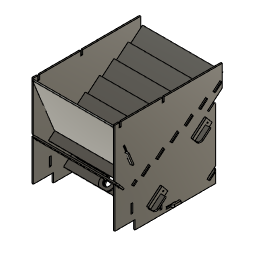
Lego Feeder (Autodesk Fusion 360 design; units mm, degrees)
Autodesk Fusion 360 part; units mm, degrees
sketch "Sketch2" plane through (0, 0, 0) normal (0, 0, 1) x (1, 0, 0) in component "SidePanel"
  line L0 (-258.4316, 256.8054) -> (-243.1107, 269.6612)
  line L1 (-243.1107, 269.6612) -> (-245.0391, 271.9593)
  line L2 (-260.36, 259.1035) -> (-245.0391, 271.9593)
  line L3 (-258.4316, 256.8054) -> (-260.36, 259.1035)
  line L4 (-228.4061, 275.4727) -> (-213.0852, 288.3285)
  line L5 (-226.4778, 273.1746) -> (-228.4061, 275.4727)
  line L6 (-211.1569, 286.0304) -> (-213.0852, 288.3285)
  line L7 (-226.4778, 273.1746) -> (-211.1569, 286.0304)
  line L8 (-164.4984, 308.2112) -> (-149.1775, 321.0669)
  line L9 (-162.5701, 305.913) -> (-164.4984, 308.2112)
  line L10 (-162.5701, 305.913) -> (-147.2492, 318.7688)
  line L11 (-147.2492, 318.7688) -> (-149.1775, 321.0669)
  line L12 (-196.4523, 291.842) -> (-181.1314, 304.6977)
  line L13 (-194.5239, 289.5438) -> (-196.4523, 291.842)
  line L14 (-179.203, 302.3996) -> (-181.1314, 304.6977)
  line L15 (-194.5239, 289.5438) -> (-179.203, 302.3996)
  line L16 (-132.5446, 324.5804) -> (-117.2237, 337.4361)
  line L17 (-130.6162, 322.2822) -> (-132.5446, 324.5804)
  line L18 (-115.2953, 335.138) -> (-117.2237, 337.4361)
  line L19 (-130.6162, 322.2822) -> (-115.2953, 335.138)
  line L20 (-100.5907, 340.9496) -> (-85.2698, 353.8053)
  line L21 (-98.6623, 338.6515) -> (-100.5907, 340.9496)
  line L22 (-83.3414, 351.5072) -> (-85.2698, 353.8053)
  line L23 (-98.6623, 338.6515) -> (-83.3414, 351.5072)
  line L24 (-320, 385) -> (-310, 385)
  line L25 (-310, 385) -> (-310, 375)
  line L26 (-310, 375) -> (-306, 375)
  line L27 (-306, 375) -> (-306, 385)
  line L28 (-214, 385) -> (-214, 375)
  line L29 (-214, 375) -> (-210, 375)
  line L30 (-210, 375) -> (-210, 385)
  line L31 (-306, 385) -> (-214, 385)
  line L32 (-210, 385) -> (-80, 385)
  line L33 (-270, 160) -> (-95, 160)
  line L34 (-270, 160) -> (-275, 160)
  line L35 (-275, 160) -> (-275, 180)
  line L36 (-320, 180) -> (-275, 180)
  line L37 (-110.3209, 306.5578) -> (-112.892, 309.6219)
  line L38 (-112.892, 309.6219) -> (-80, 337.2216)
  line L39 (-320, 270) -> (-310.3582, 258.5093)
  line L40 (-310.3582, 258.5093) -> (-307.294, 261.0805)
  line L41 (-307.294, 261.0805) -> (-320, 276.2229)
  line L42 (-110.3209, 306.5578) -> (-98.8302, 316.1996)
  arc A0 (-95, 314.5191) -> (-98.8302, 316.1996) centre (-97.3306, 314.4124) ccw
  line L43 (-245.0047, 186.3535) -> (-242.4335, 183.2893)
  line L44 (-245.0047, 186.3535) -> (-222.0233, 205.6371)
  line L45 (-242.4335, 183.2893) -> (-219.4522, 202.5729)
  line L46 (-219.4522, 202.5729) -> (-222.0233, 205.6371)
  line L47 (-122.4376, 289.1995) -> (-119.8664, 286.1353)
  line L48 (-122.4376, 289.1995) -> (-145.4189, 269.9158)
  line L49 (-119.8664, 286.1353) -> (-142.8477, 266.8517)
  line L50 (-142.8477, 266.8517) -> (-145.4189, 269.9158)
  line L51 (-80, 337.2216) -> (-80, 385)
  line L52 (-95, 160) -> (-95, 189)
  line L53 (-95, 194.2216) -> (-95, 314.5191)
  line L54 (-95, 189) -> (-106.4907, 179.3582)
  line L55 (-106.4907, 179.3582) -> (-109.0618, 182.4224)
  line L56 (-109.0618, 182.4224) -> (-95, 194.2216)
  line L57 (-272.7665, 255.2203) -> (-274.6948, 257.5184)
  line L58 (-272.7665, 255.2203) -> (-280.4269, 248.7924)
  line L59 (-274.6948, 257.5184) -> (-282.3553, 251.0906)
  line L60 (-280.4269, 248.7924) -> (-282.3553, 251.0906)
  line L61 (-320, 180) -> (-320, 270)
  line L62 (-320, 276.2229) -> (-320, 385)
  line L63 (-280, 195) -> (-284, 195)
  line L64 (-284, 195) -> (-284, 215)
  line L65 (-284, 215) -> (-280, 215)
  line L66 (-280, 215) -> (-280, 195)
  line L67 (-287.3826, 307.9489) -> (-298.1337, 335.9564)
  line L68 (-287.3826, 307.9489) -> (-290.1834, 306.8738)
  line L69 (-290.1834, 306.8738) -> (-300.9344, 334.8813)
  line L70 (-300.9344, 334.8813) -> (-298.1337, 335.9564)
  line L71 (-219, 170) -> (-219, 190)
  line L72 (-219, 190) -> (-215, 190)
  line L73 (-215, 190) -> (-215, 170)
  line L74 (-215, 170) -> (-219, 170)
  line L75 (-185, 165) -> (-205, 165)
  line L76 (-205, 165) -> (-205, 170)
  line L77 (-205, 170) -> (-185, 170)
  line L78 (-185, 170) -> (-185, 165)
  dimension "d102_1" = 20
  dimension "d107_1" = 20
  dimension "d109_1" = 20
  dimension "d111_1" = 20
  dimension "d113_1" = 20
  dimension "d115_1" = 20
  dimension "d2" = 4
  dimension "d3" = 15
  dimension "d4" = 15
  dimension "d104" = 4
  dimension "d110" = 4
  dimension "d112" = 30
  dimension "d118" = 15
  dimension "d119" = 4
  dimension "d134" = 10
  dimension "d163" = 3
  dimension "d164" = 30
  dimension "d165" = 20
  dimension "d166" = 5
  constraint perpendicular L0 L1
  constraint perpendicular L2 L3
  constraint perpendicular L6 L7
  constraint perpendicular L4 L5
  constraint perpendicular L14 L15
  constraint perpendicular L12 L13
  constraint perpendicular L10 L11
  constraint perpendicular L8 L9
  constraint perpendicular L18 L19
  constraint perpendicular L16 L17
  constraint perpendicular L22 L23
  constraint perpendicular L20 L21
  constraint perpendicular L24 L25
  constraint perpendicular L25 L26
  constraint perpendicular L27 L29
  constraint perpendicular L28 L31
  constraint perpendicular L37 L38
  constraint perpendicular L39 L40
  constraint perpendicular L40 L41
  constraint perpendicular L37 L42
  constraint tangent L42 A0
  constraint perpendicular L43 L44
  constraint perpendicular L43 L45
  constraint perpendicular L47 L48
  constraint perpendicular L47 L49
  constraint perpendicular L33 L52
  constraint perpendicular L54 L55
  constraint perpendicular L55 L56
  constraint perpendicular L57 L58
  constraint perpendicular L57 L59
  constraint perpendicular L59 L60
  constraint perpendicular L24 L62
  constraint horizontal L63
  constraint vertical L64
  constraint horizontal L65
  constraint vertical L66
  constraint perpendicular L67 L68
  constraint perpendicular L68 L69
  constraint horizontal L74
  constraint vertical L71
  constraint horizontal L72
  constraint vertical L73
  constraint horizontal L75
  constraint vertical L76
  constraint horizontal L77
  constraint vertical L78
  measures "d102_1" distance of L0.start L0.end
  measures "d107_1" distance of L6.start L5.start
  measures "d109_1" distance of L13.start L14.start
  measures "d111_1" distance of L9.start L10.end
  measures "d113_1" distance of L18.start L17.start
  measures "d115_1" distance of L21.start L22.start
  measures "d2" distance of L37.start L37.end
  measures "d3" distance of L39.start L39.end
  measures "d4" distance of L37.start L42.end
  measures "d104" distance of L43.start L43.end
  measures "d110" distance of L47.start L47.end
  measures "d112" distance of L47.end L49.end
  measures "d118" distance of L52.end L54.end
  measures "d119" distance of L54.end L55.end
  measures "d134" distance of L57.end L59.end
  measures "d163" distance of L67.start L68.end
  measures "d164" distance of L68.end L69.end
  measures "d165" distance of L75.start L75.end
  measures "d166" distance of L75.start L77.end
sketch "Sketch1" plane through (0, 0, 0) normal (0, 0, 1) x (1, 0, 0) in component "BackWall"
  line L0 (-315, 105) -> (-318, 105)
  line L1 (-315, 105) -> (-315, 55)
  line L2 (-315, 55) -> (-136, 55)
  line L3 (-136, 55) -> (-136, 105)
  line L4 (-318, 105) -> (-318, 90)
  line L5 (-315, 120) -> (-315, 185)
  line L6 (-315, 185) -> (-136, 185)
  line L7 (-136, 185) -> (-136, 120)
  line L8 (-133, 90) -> (-133, 105)
  line L9 (-133, 105) -> (-136, 105)
  line L10 (-318, 90) -> (-324, 90)
  line L11 (-324, 90) -> (-324, 120)
  line L12 (-324, 120) -> (-315, 120)
  line L13 (-133, 90) -> (-127, 90)
  line L14 (-127, 90) -> (-127, 120)
  line L15 (-127, 120) -> (-136, 120)
  dimension "d143" = 50
  dimension "d144" = 179
  dimension "d145" = 15
  dimension "d148" = 65
  constraint perpendicular L0 L1
  constraint perpendicular L2 L3
  constraint perpendicular L0 L4
  constraint perpendicular L5 L6
  constraint perpendicular L6 L7
  constraint perpendicular L4 L10
  constraint perpendicular L10 L11
  constraint perpendicular L5 L12
  constraint perpendicular L7 L15
  measures "d143" distance of L0.start L1.end
  measures "d144" distance of L1.end L2.end
  measures "d145" distance of L0.end L4.end
  measures "d148" distance of L5.start L5.end
extrude "Extrude1" add sketch "Sketch2" along normal blind 3 makes body 1 in component "SidePanel"
sketch "Sketch1 (2)" plane through (0, 0, 0) normal (0, 0, 1) x (1, 0, 0) in component "Step"
  line L0 (25, 360) -> (204, 360)
  line L1 (204, 403) -> (25, 403)
  line L2 (25, 403) -> (25, 393)
  line L3 (25, 373) -> (25, 360)
  line L4 (204, 403) -> (204, 393)
  line L5 (204, 373) -> (204, 360)
  line L6 (25, 373) -> (19, 373)
  line L7 (19, 373) -> (19, 393)
  line L8 (19, 393) -> (25, 393)
  line L9 (204, 373) -> (210, 373)
  line L10 (210, 373) -> (210, 393)
  line L11 (210, 393) -> (204, 393)
  dimension "d5" = 179
  dimension "d6" = 43
  dimension "d7" = 10
  dimension "d10" = 10
  dimension "d204" = 6
  dimension "d205" = 20
  constraint horizontal L0
  constraint horizontal L1
  constraint perpendicular L1 L2
  constraint perpendicular L1 L4
  constraint perpendicular L0 L5
  constraint perpendicular L3 L6
  constraint perpendicular L6 L7
  constraint perpendicular L9 L10
  measures "d5" distance of L0.start L0.end
  measures "d6" distance of L0.start L1.end
  measures "d7" distance of L1.end L2.end
  measures "d10" distance of L1.start L4.end
  measures "d204" distance of L3.start L6.end
  measures "d205" distance of L6.end L7.end
sketch "Sketch1 (3)" plane through (0, 0, 0) normal (0, 0, 1) x (1, 0, 0) in component "LastStep"
  line L0 (25, 423) -> (25, 410)
  line L1 (25, 410) -> (204, 410)
  line L2 (204, 423) -> (204, 410)
  line L3 (25, 443) -> (25, 448)
  line L4 (25, 448) -> (204, 448)
  line L5 (204, 448) -> (204, 443)
  line L6 (204, 423) -> (210, 423)
  line L7 (210, 423) -> (210, 443)
  line L8 (210, 443) -> (204, 443)
  line L9 (25, 423) -> (19, 423)
  line L10 (19, 423) -> (19, 443)
  line L11 (19, 443) -> (25, 443)
  dimension "d11" = 179
  dimension "d206" = 6
  constraint horizontal L1
  constraint perpendicular L1 L2
  constraint perpendicular L6 L7
  constraint perpendicular L0 L9
  measures "d11" distance of L1.end L0.end
  measures "d206" distance of L0.start L9.end
sketch "Sketch1 (4)" plane through (0, 0, 0) normal (0, 0, 1) x (1, 0, 0) in component "MovingStep"
  line L0 (26, 355) -> (203, 355)
  circle A0 centre (90, 265) radius 1.5
  circle A1 centre (139, 265) radius 1.5
  circle A2 centre (114.5, 265) radius 4
  arc A3 (146, 258) -> (153, 265) centre (146, 265) ccw
  line L1 (146, 258) -> (83, 258)
  arc A4 (76, 265) -> (83, 258) centre (83, 265) ccw
  line L2 (153, 265) -> (153, 300)
  arc A5 (160, 307) -> (153, 300) centre (160, 300) ccw
  line L3 (76, 265) -> (76, 300)
  arc A6 (76, 300) -> (69, 307) centre (69, 300) ccw
  line L4 (160, 307) -> (196, 307)
  line L5 (203, 355) -> (203, 314)
  arc A7 (196, 307) -> (203, 314) centre (196, 314) ccw
  line L6 (69, 307) -> (33, 307)
  line L7 (26, 355) -> (26, 314)
  arc A8 (26, 314) -> (33, 307) centre (33, 314) ccw
  circle A9 centre (139, 300) radius 2.6
  circle A10 centre (90, 300) radius 2.6
  circle A11 centre (114.5, 300) radius 6
  dimension "d26" = 3
  dimension "d27" = 8
  dimension "d32" = 63
  dimension "d33" = 35
  dimension "d36" = 35
  dimension "d37" = 36
  dimension "d38" = 41
  dimension "d39" = 36
  dimension "d40" = 41
  dimension "d181" = 5.2
  dimension "d182" = 5.2
  dimension "d203" = 12
  constraint horizontal L0
  constraint tangent L2 A5
  constraint vertical L3
  constraint tangent L3 A6
  constraint perpendicular L0 L5
  constraint tangent L5 A7
  constraint tangent L4 A7
  constraint perpendicular L0 L7
  constraint tangent L7 A8
  measures "d26" diameter of A1
  measures "d27" diameter of A2
  measures "d32" distance of A3.start L1.end
  measures "d33" distance of A3.end L2.end
  measures "d36" distance of A4.start L3.end
  measures "d37" distance of A5.start L4.end
  measures "d38" distance of L0.end L5.end
  measures "d39" distance of A6.end L6.end
  measures "d40" distance of L0.start L7.end
  measures "d181" diameter of A9
  measures "d182" diameter of A10
  measures "d203" diameter of A11
sketch "Sketch1 (5)" plane through (0, 0, 0) normal (0, 0, 1) x (1, 0, 0) in component "StepSpacer"
  circle A0 centre (139, 249) radius 1.5
  circle A1 centre (90, 249) radius 1.5
  circle A2 centre (114.5, 249) radius 4
  arc A3 (83, 256) -> (83, 242) centre (83, 249) ccw
  arc A4 (146, 242) -> (146, 256) centre (146, 249) ccw
  line L0 (83, 256) -> (146, 256)
  line L1 (146, 242) -> (83, 242)
  dimension "d41" = 3
  dimension "d42" = 8
  constraint tangent A4 L0
  constraint tangent A3 L1
  measures "d41" diameter of A0
  measures "d42" diameter of A2
sketch "Sketch2 (2)" plane through (0, 0, 0) normal (0, 0, 1) x (1, 0, 0) in component "MovingStepFirst"
  arc A0 (340, 307) -> (333, 300) centre (340, 300) ccw
  line L0 (383, 355) -> (383, 314)
  line L1 (249, 307) -> (213, 307)
  line L2 (340, 307) -> (376, 307)
  arc A1 (206, 314) -> (213, 307) centre (213, 314) ccw
  line L3 (206, 355) -> (206, 314)
  line L4 (206, 355) -> (383, 355)
  arc A2 (256, 300) -> (249, 307) centre (249, 300) ccw
  arc A3 (376, 307) -> (383, 314) centre (376, 314) ccw
  arc A4 (326, 293) -> (333, 300) centre (326, 300) ccw
  arc A5 (256, 300) -> (263, 293) centre (263, 300) ccw
  line L5 (263, 293) -> (326, 293)
  circle A6 centre (319, 300) radius 2.6
  circle A7 centre (270, 300) radius 2.6
  dimension "d61" = 36
  dimension "d62" = 41
  dimension "d63" = 36
  dimension "d64" = 41
  dimension "d183" = 5.2
  dimension "d184" = 5.2
  constraint horizontal L4
  constraint perpendicular L0 L4
  constraint tangent L0 A3
  constraint tangent L2 A3
  constraint perpendicular L3 L4
  constraint tangent A1 L3
  constraint tangent A4 L5
  measures "d61" distance of A0.start L2.end
  measures "d62" distance of L0.start L0.end
  measures "d63" distance of L1.start L1.end
  measures "d64" distance of A1.start L3.start
  measures "d183" diameter of A6
  measures "d184" diameter of A7
sketch "Sketch1 (6)" plane through (0, 0, 0) normal (0, 0, 1) x (1, 0, 0) in component "Brace"
  line L0 (25, 215) -> (204, 215)
  line L1 (204, 215) -> (204, 225)
  line L2 (204, 225) -> (207, 225)
  line L3 (207, 225) -> (207, 215)
  line L4 (207, 215) -> (211, 215)
  line L5 (25, 215) -> (25, 225)
  line L6 (25, 225) -> (22, 225)
  line L7 (22, 225) -> (22, 215)
  line L8 (22, 215) -> (18, 215)
  line L9 (211, 215) -> (211, 231)
  arc A0 (211, 231) -> (207, 235) centre (207, 231) ccw
  line L10 (18, 215) -> (18, 231)
  line L11 (207, 235) -> (22, 235)
  arc A1 (22, 235) -> (18, 231) centre (22, 231) ccw
  dimension "d65" = 179
  constraint horizontal L0
  constraint perpendicular L0 L1
  constraint perpendicular L1 L2
  constraint perpendicular L2 L3
  constraint perpendicular L3 L4
  constraint perpendicular L0 L5
  constraint perpendicular L5 L6
  constraint perpendicular L0 L7
  constraint perpendicular L7 L8
  constraint perpendicular L4 L9
  constraint tangent L9 A0
  constraint perpendicular L8 L10
  constraint horizontal L11
  constraint tangent L10 A1
  measures "d65" distance of L0.start L0.end
extrude "Extrude1'" add sketch "Sketch1 (4)" along normal blind 4 separate body contours L0 A3 L1 A4 L2 A5 L3 A6 L4 L5 A7 L6 L7 A8 | A11 makes body 2 in component "MovingStep"
extrude "Extrude1''" add sketch "Sketch1 (5)" along normal blind 4 separate body makes body 3 in component "StepSpacer"
extrude "Extrude1'''" add sketch "Sketch2 (2)" along normal blind 4 separate body makes body 4 in component "MovingStepFirst"
extrude "Extrude1''''" add sketch "Sketch1 (2)" along normal blind 3 separate body makes body 5 in component "Step"
extrude "Extrude1'''''" add sketch "Sketch1 (3)" along normal blind 3 separate body makes body 6 in component "LastStep"
sketch "Sketch1 (7)" plane through (0, 0, 0) normal (0, 0, 1) x (1, 0, 0) in component "Mount"
  line L0 (25, 205) -> (204, 205)
  line L1 (204, 25) -> (25, 25)
  circle A0 centre (129.5, 100) radius 1.5
  circle A1 centre (99.5, 100) radius 1.5
  circle A2 centre (99.5, 130) radius 1.5
  circle A3 centre (129.5, 130) radius 1.5
  circle A4 centre (114.5, 122) radius 6.5
  line L2 (25, 25) -> (25, 35)
  line L3 (204, 195) -> (204, 205)
  line L4 (204, 25) -> (204, 35)
  arc A5 (204, 155) -> (204, 75) centre (204, 115) ccw
  line L5 (204, 65) -> (204, 75)
  line L6 (204, 155) -> (204, 165)
  line L7 (25, 195) -> (25, 205)
  line L8 (25, 165) -> (25, 155)
  line L9 (25, 65) -> (25, 75)
  arc A6 (25, 75) -> (25, 155) centre (25, 115) ccw
  arc A7 (108, 143) -> (121, 143) centre (114.5, 143) ccw
  arc A8 (121, 192) -> (108, 192) centre (114.5, 192) ccw
  arc A9 (121, 87) -> (108, 87) centre (114.5, 87) ccw
  arc A10 (108, 38) -> (121, 38) centre (114.5, 38) ccw
  line L10 (108, 38) -> (108, 87)
  line L11 (121, 38) -> (121, 87)
  line L12 (108, 143) -> (108, 192)
  line L13 (121, 143) -> (121, 192)
  circle A11 centre (127, 84) radius 1.5
  circle A12 centre (102, 84) radius 1.5
  circle A13 centre (102, 41) radius 1.5
  circle A14 centre (127, 41) radius 1.5
  circle A15 centre (127, 146) radius 1.5
  circle A16 centre (102, 146) radius 1.5
  circle A17 centre (102, 189) radius 1.5
  circle A18 centre (127, 189) radius 1.5
  line L14 (204, 65) -> (206.8, 65)
  line L15 (206.8, 35) -> (204, 35)
  line L16 (211.2, 65) -> (211.2, 55)
  line L17 (211.2, 55) -> (206.8, 55)
  line L18 (211.2, 65) -> (221.2, 65)
  arc A19 (214.2, 35) -> (221.2, 42) centre (214.2, 42) ccw
  line L19 (206.8, 35) -> (214.2, 35)
  line L20 (221.2, 42) -> (221.2, 65)
  line L21 (206.8, 55) -> (206.8, 65)
  line L22 (221.2, 172) -> (221.2, 195)
  line L23 (211.2, 195) -> (211.2, 185)
  arc A20 (214.2, 165) -> (221.2, 172) centre (214.2, 172) ccw
  line L24 (206.8, 165) -> (214.2, 165)
  line L25 (206.8, 185) -> (206.8, 195)
  line L26 (211.2, 185) -> (206.8, 185)
  line L27 (211.2, 195) -> (221.2, 195)
  line L28 (206.8, 195) -> (204, 195)
  line L29 (206.8, 165) -> (204, 165)
  line L30 (7.8, 42) -> (7.8, 65)
  line L31 (17.8, 65) -> (17.8, 55)
  arc A21 (14.8, 35) -> (7.8, 42) centre (14.8, 42) cw
  line L32 (22.2, 35) -> (14.8, 35)
  line L33 (22.2, 55) -> (22.2, 65)
  line L34 (17.8, 55) -> (22.2, 55)
  line L35 (17.8, 65) -> (7.8, 65)
  line L36 (22.2, 65) -> (25, 65)
  line L37 (22.2, 35) -> (25, 35)
  line L38 (17.8, 65) -> (17.8, 55)
  line L39 (22.2, 55) -> (22.2, 65)
  line L40 (17.8, 55) -> (22.2, 55)
  line L41 (22.2, 35) -> (14.8, 35)
  line L42 (17.8, 65) -> (7.8, 65)
  arc A22 (14.8, 35) -> (7.8, 42) centre (14.8, 42) cw
  line L43 (7.8, 42) -> (7.8, 65)
  line L44 (17.8, 195) -> (17.8, 185)
  line L45 (22.2, 185) -> (22.2, 195)
  line L46 (17.8, 185) -> (22.2, 185)
  line L47 (22.2, 165) -> (14.8, 165)
  line L48 (17.8, 195) -> (7.8, 195)
  arc A23 (14.8, 165) -> (7.8, 172) centre (14.8, 172) cw
  line L49 (7.8, 172) -> (7.8, 195)
  line L50 (22.2, 195) -> (25, 195)
  line L51 (22.2, 165) -> (25, 165)
  dimension "d85" = 179
  dimension "d86" = 180
  dimension "d185" = 2.8
  dimension "d187" = 10
  dimension "d190" = 10
  dimension "d191" = 10
  dimension "d192" = 10
  dimension "d193" = 10
  constraint horizontal L0
  constraint horizontal L1
  constraint perpendicular L0 L3
  constraint perpendicular L0 L7
  constraint tangent A9 L10
  constraint tangent A9 L11
  constraint tangent A8 L12
  constraint perpendicular L5 L14
  constraint perpendicular L16 L18
  constraint tangent A19 L19
  constraint tangent A19 L20
  constraint perpendicular L14 L21
  constraint perpendicular L23 L27
  constraint tangent A20 L24
  constraint tangent L22 A20
  constraint perpendicular L31 L35
  constraint tangent A21 L32
  constraint tangent L30 A21
  constraint perpendicular L9 L36
  constraint perpendicular L38 L42
  constraint tangent L41 A22
  constraint tangent A22 L43
  constraint perpendicular L44 L48
  constraint tangent L47 A23
  constraint tangent A23 L49
  measures "d85" distance of L0.start L0.end
  measures "d86" distance of L0.start L1.end
  measures "d185" distance of L5.start L14.end
  measures "d187" distance of L16.start L18.end
  measures "d190" distance of L23.start L22.end
  measures "d191" distance of L31.start L30.end
  measures "d192" distance of L31.start L30.end
  measures "d193" distance of L44.start L48.end
extrude "Extrude2" add sketch "Sketch1 (7)" along normal blind 4 separate body makes body 7 in component "Mount"
sketch "Sketch1 (8)" plane through (0, 0, 0) normal (0, 0, 1) x (1, 0, 0) in component "BearingGuide"
  line L0 (242.941, 100) -> (226.059, 100)
  arc A0 (226.059, 100) -> (219, 87) centre (234.5, 87) ccw
  line L1 (219, 38) -> (219, 87)
  arc A1 (219, 38) -> (226.059, 25) centre (234.5, 38) ccw
  line L2 (226.059, 25) -> (242.941, 25)
  arc A2 (242.941, 25) -> (250, 38) centre (234.5, 38) ccw
  line L3 (250, 38) -> (250, 87)
  arc A3 (250, 87) -> (242.941, 100) centre (234.5, 87) ccw
  circle A4 centre (247, 41) radius 1.5
  circle A5 centre (222, 41) radius 1.5
  circle A6 centre (222, 84) radius 1.5
  circle A7 centre (247, 84) radius 1.5
  arc A8 (226.25, 38) -> (242.75, 38) centre (234.5, 38) ccw
  arc A9 (242.75, 87) -> (226.25, 87) centre (234.5, 87) ccw
  line L4 (226.25, 38) -> (226.25, 87)
  line L5 (242.75, 38) -> (242.75, 87)
  dimension "d196" = 8.25
  dimension "d197" = 8.25
  constraint tangent L3 A3
  constraint tangent A0 L1
  constraint coincident A0.centre A3.centre
  constraint tangent A9 L4
  constraint tangent A9 L5
  measures "d196" radius of A8
  measures "d197" radius of A9
extrude "Extrude1''''''" add sketch "Sketch1 (8)" along normal blind 3 separate body makes body 8 in component "BearingGuide"
extrude "Extrude1'''''''" add sketch "Sketch1 (6)" along normal blind 3 separate body makes body 9 in component "Brace"
sketch "Sketch2 (3)" plane through (0, 0, 0) normal (0, 0, 1) x (1, 0, 0) in component "FirstStep"
  line L0 (25, 453) -> (204, 453)
  line L1 (25, 473) -> (204, 473)
  line L2 (204, 473) -> (204, 468)
  line L3 (25, 453) -> (25, 458)
  line L4 (204, 453) -> (204, 458)
  line L5 (25, 473) -> (25, 468)
  line L6 (25, 458) -> (19, 458)
  line L7 (19, 458) -> (19, 468)
  line L8 (19, 468) -> (25, 468)
  line L9 (204, 458) -> (210, 458)
  line L10 (210, 458) -> (210, 468)
  line L11 (210, 468) -> (204, 468)
  dimension "d126" = 179
  dimension "d129" = 5
  dimension "d207" = 6
  dimension "d208" = 10
  constraint horizontal L0
  constraint perpendicular L1 L5
  constraint perpendicular L3 L6
  constraint perpendicular L6 L7
  constraint perpendicular L4 L9
  constraint perpendicular L9 L10
  measures "d126" distance of L0.end L0.start
  measures "d129" distance of L1.start L5.end
  measures "d207" distance of L3.end L6.end
  measures "d208" distance of L6.end L7.end
extrude "Extrude1''''''''" add sketch "Sketch2 (3)" along normal blind 3 separate body makes body 10 in component "FirstStep"
extrude "Extrude1'''''''''" add sketch "Sketch1" along normal blind 3 separate body makes body 11 in component "BackWall"
sketch "Sketch1 (9)" plane through (0, 0, 0) normal (0, 0, 1) x (1, 0, 0) in component "MotorArm"
  arc A0 (261.2507, 33.25) -> (264.7493, 33.25) centre (263, 31) ccw
  circle A1 centre (285.5, 31) radius 2
  arc A2 (263, 38) -> (263, 24) centre (263, 31) ccw
  arc A3 (285.5, 24) -> (285.5, 38) centre (285.5, 31) ccw
  line L0 (263, 33.25) -> (264.7493, 33.25)
  line L1 (263, 33.25) -> (261.2507, 33.25)
  line L2 (263, 38) -> (285.5, 38)
  line L3 (285.5, 24) -> (263, 24)
  constraint coincident A1.centre A3.centre
  constraint coincident A0.centre A2.centre
  constraint tangent A2 L3
sketch "Sketch1 (10)" plane through (0, 0, 0) normal (0, 0, 1) x (1, 0, 0) in component "LinkArm"
  circle A0 centre (260, 10) radius 2.25
  circle A1 centre (319.5, 10) radius 4.25
  arc A2 (260, 17) -> (260, 3) centre (260, 10) ccw
  arc A3 (319.5, 0) -> (319.5, 20) centre (319.5, 10) ccw
  line L0 (319.5, 0) -> (260, 3)
  line L1 (260, 17) -> (319.5, 20)
  dimension "d171" = 4.5
  dimension "d172" = 59.5
  dimension "d173" = 8.5
  dimension "d175" = 7
  dimension "d176" = 10
  constraint coincident A0.centre A2.centre
  constraint coincident A1.centre A3.centre
  measures "d171" diameter of A0
  measures "d172" distance of A0.centre A1.centre
  measures "d173" diameter of A1
  measures "d175" radius of A2
  measures "d176" radius of A3
extrude "Extrude1''''''''''" add sketch "Sketch1 (10)" along normal blind 4 separate body makes body 12 in component "LinkArm"
extrude "Extrude1'''''''''''" add sketch "Sketch1 (9)" along normal blind 4 separate body makes body 13 in component "MotorArm"
sketch "Sketch1 (11)" plane through (0, 0, 0) normal (0, 0, 1) x (1, 0, 0) in component "LockingPiece"
  line L0 (273, 75) -> (273, 55)
  line L1 (273, 55) -> (265, 55)
  line L2 (285, 55) -> (277, 55)
  line L3 (277, 55) -> (277, 75)
  line L4 (285, 95) -> (265, 95)
  line L5 (273, 75) -> (277, 75)
  line L6 (265, 55) -> (265, 95)
  line L7 (285, 55) -> (285, 95)
  circle A0 centre (275, 90) radius 1.5
  dimension "d200" = 3
  constraint vertical L0
  constraint horizontal L1
  constraint horizontal L2
  constraint vertical L3
  constraint horizontal L4
  constraint perpendicular L0 L5
  constraint perpendicular L4 L6
  measures "d200" diameter of A0
extrude "Extrude1''''''''''''" add sketch "Sketch1 (11)" along normal blind 4 separate body makes body 14 in component "LockingPiece"
sketch "Sketch 1" plane through (0, 0, 0) normal (0, 0, 1) x (1, 0, 0) in component "Power supply holder"
  line L0 (-71, 19) -> (-68, 19)
  line L1 (-42, -13) -> (-64, -13)
  arc A0 (-38, -9) -> (-42, -13) centre (-42, -9) cw
  arc A1 (-64, -13) -> (-68, -9) centre (-64, -9) cw
  line L2 (-68, -9) -> (-68, 10)
  circle A2 centre (-64, 38) radius 1.25
  arc A3 (-42, 42) -> (-38, 38) centre (-42, 38) cw
  arc A4 (-75, 15) -> (-71, 19) centre (-71, 15) cw
  line L3 (-68, 19) -> (-68, 38)
  line L4 (-71, 10) -> (-71, 0)
  circle A5 centre (-42, 38) radius 1.25
  line L5 (-38, 38) -> (-38, -9)
  line L6 (-64, 42) -> (-42, 42)
  arc A6 (-68, 38) -> (-64, 42) centre (-64, 38) cw
  line L7 (-68, 10) -> (-71, 10)
  line L8 (-71, 0) -> (-75, 0)
  line L9 (-75, 0) -> (-75, 15)
  circle A7 centre (-64, -9) radius 1.25
  circle A8 centre (-42, -9) radius 1.25
extrude "Extrude1'''''''''''''" add sketch "Sketch 1" along normal blind 5 separate body makes body 15 in component "Power supply holder"
component "Templates" placed x (1, 0, 0) y (0, 1, 0) z (0, 0, 1) at (0, 0, 0)
component "LegoFeeder" placed x (1, 0, 0) y (0, 1, 0) z (0, 0, 1) at (0, 0, 0)
component "SidePanel" placed x (1, 0, 0) y (0, 1, 0) z (0, 0, 1) at (0, 0, 0) in component "Templates"
component "BackWall" placed x (1, 0, 0) y (0, 1, 0) z (0, 0, 1) at (0, -50, 0) in component "Templates"
component "Step" placed x (1, 0, 0) y (0, 1, 0) z (0, 0, 1) at (0, 0, 0) in component "Templates"
component "LastStep" placed x (1, 0, 0) y (0, 1, 0) z (0, 0, 1) at (0, 0, 0) in component "Templates"
component "MovingStep" placed x (1, 0, 0) y (0, 1, 0) z (0, 0, 1) at (0, 0, 0) in component "Templates"
component "StepSpacer" placed x (1, 0, 0) y (0, 1, 0) z (0, 0, 1) at (0, 0, 0) in component "Templates"
component "MovingStepFirst" placed x (1, 0, 0) y (0, 1, 0) z (0, 0, 1) at (0, 0, 0) in component "Templates"
component "Brace" placed x (1, 0, 0) y (0, 1, 0) z (0, 0, 1) at (0, 0, 0) in component "Templates"
component "Mount" placed x (1, 0, 0) y (0, 1, 0) z (0, 0, 1) at (0, 0, 0) in component "Templates"
component "BearingGuide" placed x (1, 0, 0) y (0, 1, 0) z (0, 0, 1) at (0, 0, 0) in component "Templates"
component "FirstStep" placed x (1, 0, 0) y (0, 1, 0) z (0, 0, 1) at (0, 0, 0) in component "Templates"
component "MotorArm" placed x (1, 0, 0) y (0, 1, 0) z (0, 0, 1) at (0, 0, 0) in component "Templates"
component "LinkArm" placed x (1, 0, 0) y (0, 1, 0) z (0, 0, 1) at (0, 0, 0) in component "Templates"
component "LockingPiece" placed x (1, 0, 0) y (0, 1, 0) z (0, 0, 1) at (0, 0, 0) in component "Templates"
component "MovingSteps" placed x (1, 0, 0) y (0, 0.766044, 0.642788) z (0, -0.642788, 0.766044) at (-77, 59.9478, 267.856) in component "LegoFeeder"
component "SidePanel" placed x (0, 1, 0) y (0, 0, 1) z (1, 0, 0) at (-54.8382, 61.6389, -156.8007) in component "LegoFeeder"
component "Steps" placed x (1, 0, 0) y (0, 1, 0) z (0, 0, 1) at (-77, 177, 95) in component "LegoFeeder"
component "Mount" placed x (1, 0, 0) y (0, 0.766044, 0.642788) z (0, -0.642788, 0.766044) at (-76.9, -207.3266, 4.075) in component "LegoFeeder"
component "BearingGuide" placed x (1, 0, 0) y (0, 0.766044, 0.642788) z (0, -0.642788, 0.766044) at (-197, -209.8432, 7.1873) in component "LegoFeeder"
component "BearingGuide" placed x (1, 0, 0) y (0, 0.766044, 0.642788) z (0, -0.642788, 0.766044) at (-197, -129.4085, 74.68) in component "LegoFeeder"
component "FirstStep" placed x (1, 0, 0) y (0, 0.766044, 0.642788) z (0, -0.642788, 0.766044) at (-76.8, -569.6873, -202.4635) in component "LegoFeeder"
component "BackWall" placed x (1, 0, 0) y (0, -0.374607, 0.927184) z (0, -0.927184, -0.374607) at (263, -187.8251, 53.7068) in component "LegoFeeder"
component "LockingPiece" placed x (0, -0.642788, 0.766044) y (0, 0.766044, 0.642788) z (-1, 0, 0) at (-55, -46.9125, -217.9663) in component "LegoFeeder"
component "SidePanel" placed x (0, 1, 0) y (0, 0, 1) z (1, 0, 0) at (127.1618, 61.6389, -156.8007) in component "LegoFeeder"
component "LockingPiece" placed x (0, 0.642788, -0.766044) y (0, 0.766044, 0.642788) z (1, 0, 0) at (131, -301.8948, 287.3274) in component "LegoFeeder"
component "LockingPiece" placed x (0, 0.642788, -0.766044) y (0, 0.766044, 0.642788) z (1, 0, 0) at (131, -400.7145, 204.4078) in component "LegoFeeder"
component "Brace" placed x (1, 0, 0) y (0, 0.766044, 0.642788) z (0, -0.642788, 0.766044) at (-77, -215.0219, -119.5512) in component "LegoFeeder"
component "Brace" placed x (1, 0, 0) y (0, -0.642788, 0.766044) z (0, -0.766044, -0.642788) at (-77, -103.2437, -65.2866) in component "LegoFeeder"
component "Power supply holder" placed x (1, 0, 0) y (0, 1, 0) z (0, 0, 1) at (0, 0, 0) in component "LegoFeeder"
component "MovingStepFirst" placed x (1, 0, 0) y (0, 1, 0) z (0, 0, 1) at (-180, -625, 40) in component "MovingSteps"
component "MovingStep" placed x (1, 0, 0) y (0, 1, 0) z (0, 0, 1) at (0, -450, 0) in component "MovingSteps"
component "MovingStep" placed x (1, 0, 0) y (0, 1, 0) z (0, 0, 1) at (0, -520, 16) in component "MovingSteps"
component "StepSpacer" placed x (1, 0, 0) y (0, 1, 0) z (0, 0, 1) at (0, -539, 28) in component "MovingSteps"
component "MovingStep" placed x (1, 0, 0) y (0, 1, 0) z (0, 0, 1) at (0, -590, 32) in component "MovingSteps"
component "MovingStep" placed x (1, 0, 0) y (0, 1, 0) z (0, 0, 1) at (0, -555, 24) in component "MovingSteps"
component "StepSpacer" placed x (1, 0, 0) y (0, 1, 0) z (0, 0, 1) at (0, -574, 36) in component "MovingSteps"
component "StepSpacer" placed x (1, 0, 0) y (0, 1, 0) z (0, 0, 1) at (0, -469, 12) in component "MovingSteps"
component "StepSpacer" placed x (1, 0, 0) y (0, 1, 0) z (0, 0, 1) at (0, -504, 20) in component "MovingSteps"
component "MovingStep" placed x (1, 0, 0) y (0, 1, 0) z (0, 0, 1) at (0, -485, 8) in component "MovingSteps"
component "StepSpacer" placed x (1, 0, 0) y (0, 1, 0) z (0, 0, 1) at (0, -434, 4) in component "MovingSteps"
component "Step" placed x (1, 0, 0) y (0, 0.766044, 0.642788) z (0, -0.642788, 0.766044) at (0, -659.7742, -234.8933) in component "Steps"
component "Step" placed x (1, 0, 0) y (0, 0.766044, 0.642788) z (0, -0.642788, 0.766044) at (0, -627.8204, -218.5241) in component "Steps"
component "Step" placed x (1, 0, 0) y (0, 0.766044, 0.642788) z (0, -0.642788, 0.766044) at (0, -595.8665, -202.1549) in component "Steps"
component "Step" placed x (1, 0, 0) y (0, 0.766044, 0.642788) z (0, -0.642788, 0.766044) at (0, -563.9126, -185.7857) in component "Steps"
component "Step" placed x (1, 0, 0) y (0, 0.766044, 0.642788) z (0, -0.642788, 0.766044) at (0, -531.9588, -169.4165) in component "Steps"
component "LastStep" placed x (1, 0, 0) y (0, 0.766044, 0.642788) z (0, -0.642788, 0.766044) at (0, -538.1342, -185.0165) in component "Steps"
